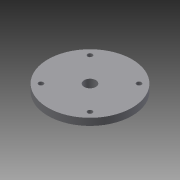
# Autodesk Inventor part: Spool Boss
Saved by Autodesk Inventor 2013 (Build 170138000, 138)
## iProperties
Created: 2013-08-04
Part Number: Spool Boss
Material: Generic
Document SubType Name: Modeling
Designer: Enlightx
Density: 1 g/cm^3
Author: Enlightx
Autodesk Inventor part; units mm, degrees
ref_plane "YZ Plane" through (0, 0, 0) normal (1, 0, 0) x (0, 1, 0)
ref_plane "XZ Plane" through (0, 0, 0) normal (0, 1, 0) x (-1, 0, 0)
ref_plane "XY Plane" through (0, 0, 0) normal (0, 0, 1) x (1, 0, 0)
sketch "Sketch1" plane through (0, 0, 0) normal (0, 0, 1) x (1, 0, 0)
  circle A0 centre (0, 0) radius 30
  dimension "d0" = 60
  constraints: 1 centre point, 1 coincident
  measures "d0" diameter of A0
extrude "Main Body" add sketch "Sketch1" along normal blind 5
sketch "Sketch7" plane through (0, 0, 0) normal (0, 0, -1) x (-1, 0, 0)
  circle A0 centre (0, 0) radius 30 projected
  circle A1 centre (0, 0) radius 10
  dimension "d32" = 20
  constraints: 1 centre point, 1 coincident
  measures "d32" diameter of A1
extrude "Raised Centre" add sketch "Sketch7" along normal blind 3 contours A1
sketch "Sketch8" plane through (0, 0, -3) normal (0, 0, -1) x (-1, 0, 0)
  circle A0 centre (0, 0) radius 10 projected
  constraints: 1 coincident
hole "Centre Hole" at (0, 0, -3) direction (0, 0, 1) diameter 8.4 end through all
sketch "Sketch10" plane through (0, 0, 0) normal (0, 0, -1) x (-1, 0, 0)
  circle A0 centre (0, 0) radius 30 projected
  line L0 (-17.5, 17.5) -> (17.5, 17.5) construction
  line L1 (17.5, 17.5) -> (17.5, -17.5) construction
  line L2 (17.5, -17.5) -> (-17.5, -17.5) construction
  line L3 (-17.5, -17.5) -> (-17.5, 17.5) construction
  line L4 (-17.5, 17.5) -> (17.5, -17.5) construction
  line L5 (17.5, 17.5) -> (-17.5, -17.5) construction
  dimension "d55" = 35
  dimension "d56" = 35
  constraints: 12 end point, 4 coincident, 2 midpoint, 2 parallel, 1 horizontal, 1 perpendicular
  measures "d55" distance of L1.end L2.end
  measures "d56" distance of L0.end L1.end
hole "Mount Holes" at (17.5, 17.5, 0) at (-17.5, 17.5, 0) at (-17.5, -17.5, 0) at (17.5, -17.5, 0) direction (0, 0, 1) diameter 3.4 end through all
sketch "Sketch11" plane through (0, 0, 0) normal (0, 0, -1) x (-1, 0, 0)
  circle A0 centre (17.5, -17.5) radius 1.7 projected
  circle A1 centre (-17.5, 17.5) radius 1.7 projected
  circle A2 centre (17.5, 17.5) radius 1.7 projected
  circle A3 centre (-17.5, -17.5) radius 1.7 projected
  line L0 (-15.9008, 14.6569) -> (-19.1627, 14.6935)
  line L1 (-19.1627, 14.6935) -> (-20.7618, 17.5367)
  line L2 (-20.7618, 17.5367) -> (-19.0992, 20.3431)
  line L3 (-19.0992, 20.3431) -> (-15.8373, 20.3065)
  line L4 (-15.8373, 20.3065) -> (-14.2382, 17.4633)
  line L5 (-14.2382, 17.4633) -> (-15.9008, 14.6569)
  line L6 (19.0992, 14.6569) -> (15.8373, 14.6935)
  line L7 (15.8373, 14.6935) -> (14.2382, 17.5367)
  line L8 (14.2382, 17.5367) -> (15.9008, 20.3431)
  line L9 (15.9008, 20.3431) -> (19.1627, 20.3065)
  line L10 (19.1627, 20.3065) -> (20.7618, 17.4633)
  line L11 (20.7618, 17.4633) -> (19.0992, 14.6569)
  line L12 (-15.8575, -20.3184) -> (-19.1195, -20.3316)
  line L13 (-19.1195, -20.3316) -> (-20.762, -17.5132)
  line L14 (-20.762, -17.5132) -> (-19.1425, -14.6816)
  line L15 (-19.1425, -14.6816) -> (-15.8805, -14.6684)
  line L16 (-15.8805, -14.6684) -> (-14.238, -17.4868)
  line L17 (-14.238, -17.4868) -> (-15.8575, -20.3184)
  line L18 (19.1425, -20.3184) -> (15.8805, -20.3316)
  line L19 (15.8805, -20.3316) -> (14.238, -17.5132)
  line L20 (14.238, -17.5132) -> (15.8575, -14.6816)
  line L21 (15.8575, -14.6816) -> (19.1195, -14.6684)
  line L22 (19.1195, -14.6684) -> (20.762, -17.4868)
  line L23 (20.762, -17.4868) -> (19.1425, -20.3184)
  dimension "d64" = 5.65
  dimension "d65" = 5.65
  dimension "d66" = 5.65
  dimension "d67" = 5.65
  constraints: 48 end point, 4 coincident, 52 other
  measures "d64" distance between parallel lines of L0 L3
  measures "d65" distance between parallel lines of L6 L9
  measures "d66" distance between parallel lines of L18 L21
  measures "d67" distance between parallel lines of L12 L15
extrude "Nut Traps" cut sketch "Sketch11" against normal blind 2.8
body "Solid1"
